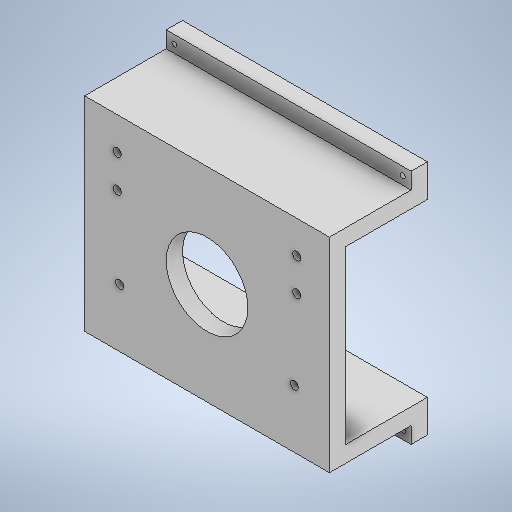
# Autodesk Inventor part: WheelCorver
Saved by Autodesk Inventor 2025.3 (Build 293356000, 356)
## iProperties
Created: 2025-04-27
Part Number: WheelCorver
Material: 일반
Document SubType Name: Modeling
Designer: SEON
Density: 1 g/cm^3
Appearance: 기본값
Author: SEON
Autodesk Inventor part; units mm, degrees
ref_plane "YZ Plane" through (0, 0, 0) normal (1, 0, 0) x (0, 1, 0)
ref_plane "XZ Plane" through (0, 0, 0) normal (0, 1, 0) x (-1, 0, 0)
ref_plane "XY Plane" through (0, 0, 0) normal (0, 0, 1) x (1, 0, 0)
sketch "스케치1" plane through (0, 0, 0) normal (0, 0, 1) x (1, 0, 0)
  line L0 (0, 0) -> (150, 0)
  line L1 (150, 0) -> (150, -145)
  line L2 (150, -145) -> (0, -145)
  line L3 (0, -145) -> (0, 0)
  line L4 (0, -20) -> (150, -20)
  line L5 (0, -125) -> (150, -125)
  line L6 (150, -135) -> (0, -135)
  line L7 (150, -10) -> (0, -10)
  circle A0 centre (21.5, -99.25) radius 2.5
  line L8 (75, -145) -> (75, -139.9922)
  circle A1 centre (128.5, -99.25) radius 2.5
  circle A2 centre (5, -5) radius 1.5
  circle A3 centre (145, -5) radius 1.5
  circle A4 centre (5, -140) radius 1.5
  circle A5 centre (145, -140) radius 1.5
  dimension "d0" = 150
  dimension "d1" = 145
  dimension "d2" = 20
  dimension "d3" = 20
  dimension "d8" = 10
  dimension "d9" = 10
  dimension "d21" = 45.75
  dimension "d22" = 21.5
  dimension "d23" = 5
  dimension "d24" = 3
  dimension "d25" = 5
  dimension "d26" = 5
  dimension "d27" = 5
  dimension "d28" = 5
  dimension "d29" = 5
  constraints: 18 end point, 8 point on line, 6 centre point, 5 perpendicular, 3 equal radius, 2 parallel, 2 vertical alignment, 1 horizontal, 1 horizontal alignment, 1 midpoint, 1 symmetric about line, 1 vertical, 1 other
  measures "d0" distance of L0.start L0.end
  measures "d1" distance of L2.end L0.start
  measures "d2" distance between parallel lines of L2 L5
  measures "d3" distance between parallel lines of L0 L4
  measures "d8" distance between parallel lines of L2 L6
  measures "d9" distance between parallel lines of L7 L4
  measures "d21" distance from line of L2 A0.centre
  measures "d22" distance from line of L3 A0.centre
  measures "d23" diameter of A0
  measures "d24" diameter of A3
  measures "d25" distance from line of L0 A2.centre
  measures "d26" distance from line of L3 A2.centre
  measures "d27" distance from line of L1 A3.centre
  measures "d28" distance from line of L0 A3.centre
  measures "d29" distance from line of L2 A5.centre
extrude "돌출1" add sketch "스케치1" along normal blind 10 contours L7 L1 L4 L3 | L4 L1 L5 L3 | L5 L1 L6 L3
extrude "돌출2" add sketch "스케치1" against normal blind 50 contours L0 L1 L7 L3 | L7 L1 L4 L3 | L5 L1 L6 L3 | L6 L1 L2 L3 | A2 | A3 | A4 | A5
extrude "돌출3" cut sketch "스케치1" against normal blind 40 contours L0 L1 L7 L3 | L6 L1 L2 L3 | A2 | A3 | A4 | A5
sketch "스케치2" plane through (0, 0, 10) normal (0, 0, 1) x (1, 0, 0)
  circle A0 centre (20, -30) radius 2.5
  circle A1 centre (130, -30) radius 2.5
  line L0 (150, -135) -> (150, -10) projected
  line L1 (0, -10) -> (0, -135) projected
  line L2 (0, 0) -> (150, 0) projected
  circle A2 centre (20, -50) radius 2.5
  circle A3 centre (130, -50) radius 2.5
  circle A4 centre (75, -72.5) radius 25
  point P0 (0, -72.5)
  point P1 (0, -72.5)
  point P2 (75, 0)
  dimension "d14" = 20
  dimension "d15" = 20
  dimension "d16" = 5
  dimension "d17" = 30
  dimension "d18" = 5
  dimension "d19" = 20
  dimension "d20" = 50
  constraints: 5 centre point, 3 horizontal alignment, 3 midpoint, 3 vertical alignment, 2 equal radius
  measures "d14" distance from line of L0 A1.centre
  measures "d15" horizontal distance of point (0, -72.5) A0.centre
  measures "d16" diameter of A0
  measures "d17" distance from line of L2 A0.centre
  measures "d18" diameter of A2
  measures "d19" distance of A1.centre A3.centre
  measures "d20" diameter of A4
extrude "돌출4" cut sketch "스케치2" against normal through all
extrude "돌출5" cut sketch "스케치1" against normal through all contours A2 | A3 | A4 | A5
equation "\"d8\" = 0.5 * d2"
equation "\"d9\" = d8"
equation "\"d25\" = 0.5 * d9"
equation "\"d26\" = d25"
equation "\"d27\" = d25"
equation "\"d28\" = d25"
equation "\"d29\" = d27"
